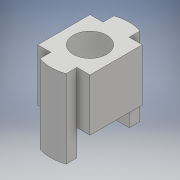
# Autodesk Inventor part: PotHandle
Saved by Autodesk Inventor 2018 (Build 220112000, 112)
## iProperties
Created: 2019-07-18
Part Number: PotHandle
Material: Generic
Document SubType Name: Modeling
Designer: aal_9
Density: 1 g/cm^3
Appearance: Default
Author: aal_9
Autodesk Inventor part; units mm, degrees
ref_plane "YZ Plane" through (0, 0, 0) normal (1, 0, 0) x (0, 1, 0)
ref_plane "XZ Plane" through (0, 0, 0) normal (0, 1, 0) x (-1, 0, 0)
ref_plane "XY Plane" through (0, 0, 0) normal (0, 0, 1) x (1, 0, 0)
sketch "Sketch1" plane through (0, 0, 0) normal (0, 0, 1) x (1, 0, 0)
  line L0 (5, 5) -> (5, -5)
  line L1 (-5, -5) -> (-5, 5)
  line L2 (5, 5) -> (-5, 5)
  line L3 (5, -5) -> (-5, -5)
  point P0 (0, 0)
  dimension "d16" = 10
  dimension "d17" = 10
  dimension "d18" = 5
  dimension "d19" = 5
  constraints: 8 end point, 2 parallel, 1 horizontal
  measures "d16" distance of L0.start L0.end
  measures "d17" distance of L0.start L1.end
  measures "d18" distance from line of point (0, 0) L2
  measures "d19" distance from line of point (0, 0) L0
extrude "Extrusion1" add sketch "Sketch1" along normal blind 10
sketch "Sketch3" plane through (0, 0, 10) normal (0, 0, 1) x (1, 0, 0)
  circle A0 centre (0, 0) radius 3.2
  dimension "d13" = 6.4
  constraints: 1 centre point, 1 coincident
  measures "d13" diameter of A0
extrude "Extrusion3" cut sketch "Sketch3" against normal up to next
sketch "Sketch4" plane through (0, 0, 10) normal (0, 0, 1) x (1, 0, 0)
  arc A0 (-2.5, -7.0711) -> (2.5, -7.0711) centre (0, 0) ccw
  arc A1 (2.5, 7.0711) -> (-2.5, 7.0711) centre (0, 0) ccw
  line L0 (5, 5) -> (-5, 5) projected
  line L1 (-5, -5) -> (5, -5) projected
  line L2 (-2.5, 5) -> (2.5, 5)
  line L3 (2.5, -5) -> (-2.5, -5)
  line L4 (-2.5, 7.0711) -> (-2.5, 5)
  line L5 (-2.5, -5) -> (-2.5, -7.0711)
  line L6 (2.5, -7.0711) -> (2.5, -5)
  line L7 (2.5, 5) -> (2.5, 7.0711)
  constraints: 12 end point, 5 parallel, 4 point on circle, 2 centre point, 2 point on line, 1 coincident, 1 horizontal
extrude "Extrusion4" add sketch "Sketch4" against normal blind 15
equation "\"d18\" = 0.5 * d16"
equation "\"d19\" = 0.5 * d17"
body "Solid1"
